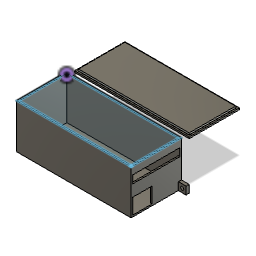
Sprinkler Case v5 (Autodesk Fusion 360 design; units mm, degrees)
Autodesk Fusion 360 part; units mm, degrees
sketch "Sketch1" plane through (0, 0, 0) normal (0, 1, 0) x (1, 0, 0)
  line L0 (0, 0) -> (145, 0)
  line L1 (0, 0) -> (0, -58)
  line L2 (0, -58) -> (145, -58)
  line L3 (145, -58) -> (145, 0)
  line L4 (145, 0) -> (0, 0)
  line L5 (0, 0) -> (0, -58)
  line L6 (0, 0) -> (-1.5, 0)
  line L7 (-1.5, 0) -> (-1.5, 1.5)
  line L8 (-1.5, 1.5) -> (0, 1.5)
  line L9 (0, 1.5) -> (0, 0)
  line L10 (145, -58) -> (146.5, -58)
  line L11 (146.5, -58) -> (146.5, -59.5)
  line L12 (146.5, -59.5) -> (145, -59.5)
  line L13 (145, -59.5) -> (145, -58)
  line L14 (-1.5, 1.5) -> (146.5, 1.5)
  line L15 (146.5, 1.5) -> (146.5, -59.5)
  line L16 (146.5, -59.5) -> (-1.5, -59.5)
  line L17 (-1.5, -59.5) -> (-1.5, 1.5)
  line L18 (146.5, 1.5) -> (148.5, 1.5)
  line L19 (148.5, 1.5) -> (148.5, 3.5)
  line L20 (148.5, 3.5) -> (146.5, 3.5)
  line L21 (146.5, 3.5) -> (146.5, 1.5)
  line L22 (-1.5, -59.5) -> (-3.5, -59.5)
  line L23 (-3.5, -59.5) -> (-3.5, -61.5)
  line L24 (-3.5, -61.5) -> (-1.5, -61.5)
  line L25 (-1.5, -61.5) -> (-1.5, -59.5)
  line L26 (-3.5, -61.5) -> (148.5, -61.5)
  line L27 (148.5, -61.5) -> (148.5, 3.5)
  line L28 (148.5, 3.5) -> (-3.5, 3.5)
  line L29 (-3.5, 3.5) -> (-3.5, -61.5)
  dimension "d7" = 145
  dimension "d8" = 58
  dimension "d9" = 1.5
  dimension "d10" = 1.5
  dimension "d11" = 1.5
  dimension "d12" = 1.5
  dimension "d13" = 2
  dimension "d14" = 2
  dimension "d15" = 2
  dimension "d16" = 2
  constraint coincident L0.start L1.start
  constraint horizontal L0
  constraint perpendicular L0 L1
  constraint horizontal L2
  constraint vertical L3
  constraint horizontal L4
  constraint vertical L5
  constraint horizontal L6
  constraint vertical L7
  constraint horizontal L8
  constraint vertical L9
  constraint horizontal L10
  constraint vertical L11
  constraint horizontal L12
  constraint vertical L13
  constraint horizontal L14
  constraint vertical L15
  constraint horizontal L16
  constraint vertical L17
  constraint horizontal L18
  constraint vertical L19
  constraint horizontal L20
  constraint vertical L21
  constraint horizontal L22
  constraint vertical L23
  constraint horizontal L24
  constraint vertical L25
  constraint horizontal L26
  constraint vertical L27
  constraint horizontal L28
  constraint vertical L29
  measures "d7" distance of L0.start L0.end
  measures "d8" distance of L0.start L1.end
  measures "d9" distance of L0.start L6.end
  measures "d10" distance of L0.start L8.end
  measures "d11" distance of L2.end L10.end
  measures "d12" distance of L2.end L12.end
  measures "d13" distance of L14.end L18.end
  measures "d14" distance of L14.end L20.end
  measures "d15" distance of L16.end L22.end
  measures "d16" distance of L16.end L24.end
extrude "Extrude1" add sketch "Sketch1" against normal blind 2 makes body 1
extrude "Extrude2" add sketch "Sketch1" along normal blind 55 contours L7 L8 L14 L17 L21 L22 L28 L29 | L22 L23 L24 L25 L26 L29 | L11 L12 L15 L16 L18 L25 L26 L27 | L18 L19 L20 L21 L27 L28 bodies 1
sketch "Sketch2" plane through (148.5, 0, 0) normal (1, 0, 0) x (0, 0, -1)
  line L0 (0, 0) -> (3.5, 0)
  line L1 (3.5, 0) -> (3.5, -2)
  line L2 (3.5, -2) -> (0, -2)
  line L3 (0, -2) -> (0, 0)
  line L4 (3.5, -2) -> (-61.5, -2)
  line L5 (-61.5, -2) -> (-61.5, 55)
  line L6 (-61.5, 55) -> (3.5, 55)
  line L7 (3.5, 55) -> (3.5, -2)
  line L8 (3.5, -2) -> (-61.5, -2)
  line L9 (-61.5, -2) -> (-61.5, 0)
  line L10 (-61.5, 0) -> (3.5, 0)
  line L11 (3.5, 0) -> (3.5, -2)
  line L12 (3.5, -2) -> (1.5, -2)
  line L13 (1.5, -2) -> (1.5, 55)
  line L14 (1.5, 55) -> (3.5, 55)
  line L15 (3.5, 55) -> (3.5, -2)
  line L16 (-61.5, -2) -> (-59.5, -2)
  line L17 (-59.5, -2) -> (-59.5, 55)
  line L18 (-59.5, 55) -> (-61.5, 55)
  line L19 (-61.5, 55) -> (-61.5, -2)
  line L20 (-59.5, 0) -> (-34.5, 0)
  line L21 (-34.5, 0) -> (-34.5, 20)
  line L22 (-34.5, 20) -> (-59.5, 20)
  line L23 (-59.5, 20) -> (-59.5, 0)
  line L24 (-59.5, 0) -> (-59.5, 45)
  line L25 (-59.5, 45) -> (1.5, 45)
  line L26 (1.5, 45) -> (1.5, 55)
  line L27 (1.5, 55) -> (-59.5, 55)
  line L28 (-59.5, 55) -> (-59.5, 45)
  line L29 (-59.5, 45) -> (1.5, 45)
  line L30 (1.5, 45) -> (1.5, 35)
  line L31 (1.5, 35) -> (-59.5, 35)
  line L32 (-59.5, 35) -> (-59.5, 45)
  dimension "d21" = 3.5
  dimension "d22" = 2
  dimension "d23" = 65
  dimension "d24" = 57
  dimension "d25" = 65
  dimension "d26" = 2
  dimension "d27" = 2
  dimension "d28" = 57
  dimension "d29" = 2
  dimension "d30" = 57
  dimension "d31" = 25
  dimension "d32" = 20
  dimension "d33" = 45
  dimension "d34" = 10
  constraint horizontal L0
  constraint vertical L1
  constraint horizontal L2
  constraint vertical L3
  constraint coincident L0.start L3.end
  constraint horizontal L4
  constraint vertical L5
  constraint horizontal L6
  constraint vertical L7
  constraint horizontal L8
  constraint vertical L9
  constraint horizontal L10
  constraint vertical L11
  constraint horizontal L12
  constraint vertical L13
  constraint horizontal L14
  constraint vertical L15
  constraint horizontal L16
  constraint vertical L17
  constraint horizontal L18
  constraint vertical L19
  constraint horizontal L20
  constraint vertical L21
  constraint horizontal L22
  constraint vertical L23
  constraint coincident L10 L20.start
  constraint coincident L17 L20.start
  constraint perpendicular L10 L24
  constraint horizontal L25
  constraint vertical L26
  constraint horizontal L27
  constraint vertical L28
  constraint horizontal L29
  constraint vertical L30
  constraint horizontal L31
  constraint vertical L32
  constraint coincident L13 L30.end
  measures "d21" distance of L0.start L0.end
  measures "d22" distance of L0.start L2.end
  measures "d23" distance of L1.end L4.end
  measures "d24" distance of L1.end L6.end
  measures "d25" distance of L1.end L4.end
  measures "d26" distance of L1.end L0.end
  measures "d27" distance of L1.end L12.end
  measures "d28" distance of L1.end L6.end
  measures "d29" distance of L4.end L16.end
  measures "d30" distance of L4.end L5.end
  measures "d31" distance of L20.start L20.end
  measures "d32" distance of L20.start L22.end
  measures "d33" distance of L20.start L24.end
  measures "d34" distance of L24.end L31.end
extrude "Extrude3" cut sketch "Sketch2" against normal blind 2 contours L10 L17 L20 L21 L22 L23 L24 | L13 L17 L24 L25 L29 L30 L31 L32 bodies 1
split "Split1" by plane through (146.5, 0, -1.5) normal (-1, 0, 0) bodies 1 makes body 2 at (96.5, -2, 39.8333)
ref_plane "WorkPlane1" through (142.5, 26.5, 29) normal (-1, 0, 0) x (0, 0, 1)
split "Split2" by plane through (142.5, 26.5, 29) normal (-1, 0, 0) bodies 2 makes body 3 at (93.8333, -2, 39.8333)
move_body "Move1" bodies 2 to x (1, 0, 0) y (0, 1, 0) z (0, 0, 1) at (0, 0, 85)
move_body "Move2" bodies 1 to x (1, 0, 0) y (0, 1, 0) z (0, 0, 1) at (-4, 0, 0)
combine "Combine1" operation add target body 3 tool bodies 1
sketch "Sketch3" plane through (0, 55, 0) normal (0, 1, 0) x (-1, 0, 0)
  line L0 (0, 0) -> (3.5, 0)
  line L1 (3.5, 0) -> (3.5, -3.5)
  line L2 (3.5, -3.5) -> (0, -3.5)
  line L3 (0, -3.5) -> (0, 0)
  line L4 (0, 0) -> (1.5, 0)
  line L5 (1.5, 0) -> (1.5, -1.5)
  line L6 (1.5, -1.5) -> (0, -1.5)
  line L7 (0, -1.5) -> (0, 0)
  line L8 (1.5, -1.5) -> (-142.5, -1.5)
  line L9 (-142.5, -1.5) -> (-142.5, 59.5)
  line L10 (-142.5, 59.5) -> (1.5, 59.5)
  line L11 (1.5, 59.5) -> (1.5, -1.5)
  line L12 (-142.5, 59.5) -> (-144.5, 59.5)
  line L13 (-144.5, 59.5) -> (-144.5, 61.5)
  line L14 (-144.5, 61.5) -> (-142.5, 61.5)
  line L15 (-142.5, 61.5) -> (-142.5, 59.5)
  line L16 (3.5, -3.5) -> (-144.5, -3.5)
  line L17 (-144.5, -3.5) -> (-144.5, 61.5)
  line L18 (-144.5, 61.5) -> (3.5, 61.5)
  line L19 (3.5, 61.5) -> (3.5, -3.5)
  dimension "d38" = 3.5
  dimension "d39" = 3.5
  dimension "d40" = 144
  dimension "d41" = 61
  dimension "d42" = 2
  dimension "d43" = 2
  constraint horizontal L0
  constraint vertical L1
  constraint horizontal L2
  constraint vertical L3
  constraint coincident L0.start L3.end
  constraint horizontal L4
  constraint vertical L5
  constraint horizontal L6
  constraint vertical L7
  constraint horizontal L8
  constraint vertical L9
  constraint horizontal L10
  constraint vertical L11
  constraint horizontal L12
  constraint vertical L13
  constraint horizontal L14
  constraint vertical L15
  constraint horizontal L16
  constraint vertical L17
  constraint horizontal L18
  constraint vertical L19
  measures "d38" distance of L0.start L0.end
  measures "d39" distance of L0.start L2.end
  measures "d40" distance of L5.end L8.end
  measures "d41" distance of L5.end L10.end
  measures "d42" distance of L9.end L12.end
  measures "d43" distance of L9.end L14.end
extrude "Extrude4" add sketch "Sketch3" along normal blind 2 separate body makes body 4
extrude "Extrude5" add sketch "Sketch3" against normal blind 2 separate body contours L0 L3 L4 L7 L8 L9 L10 L11 | L0 L3 L4 L5 L6 L7 L8 L11 makes body 5
combine "Combine2" operation add target body 4 tool bodies 5
chamfer "Chamfer1" distance 0.5 distance2 1.75 1 faces at (46.5, 53, 18.8333) on bodies 4
sketch "Sketch4" plane through (144.5, 0, 0) normal (1, 0, 0) x (0, 0, -1)
  line L0 (3.5, -2) -> (-0.5, -2)
  line L1 (-0.5, -2) -> (-0.5, 8)
  line L2 (-0.5, 8) -> (3.5, 8)
  line L3 (3.5, 8) -> (3.5, -2)
  dimension "d50" = 4
  dimension "d51" = 10
  constraint horizontal L0
  constraint vertical L1
  constraint horizontal L2
  constraint vertical L3
  measures "d50" distance of L0.start L0.end
  measures "d51" distance of L0.start L2.end
extrude "Extrude6" add sketch "Sketch4" along normal blind 10 bodies 3
sketch "Sketch5" plane through (-3.5, 0, 0) normal (-1, 0, 0) x (0, 0, 1)
  line L0 (-3.5, -2) -> (0.5, -2)
  line L1 (0.5, -2) -> (0.5, 8)
  line L2 (0.5, 8) -> (-3.5, 8)
  line L3 (-3.5, 8) -> (-3.5, -2)
  dimension "d54" = 4
  dimension "d55" = 10
  constraint horizontal L0
  constraint vertical L1
  constraint horizontal L2
  constraint vertical L3
  measures "d54" distance of L0.start L0.end
  measures "d55" distance of L0.start L2.end
extrude "Extrude7" add sketch "Sketch5" along normal blind 10 bodies 3
sketch "Sketch6" plane through (0, 0, 0.5) normal (0, 0, 1) x (1, 0, 0)
  line L0 (-3.5, -2) -> (-13.5, -2)
  line L1 (-13.5, -2) -> (-13.5, 8)
  line L2 (-13.5, 8) -> (-3.5, 8)
  line L3 (-3.5, 8) -> (-3.5, -2)
  line L4 (-3.5, -2) -> (-8.5, -2)
  line L5 (-8.5, -2) -> (-8.5, 3)
  line L6 (-8.5, 3) -> (-3.5, 3)
  line L7 (-3.5, 3) -> (-3.5, -2)
  circle A0 centre (-8.5, 3) radius 2
  dimension "d58" = 10
  dimension "d59" = 10
  dimension "d60" = 5
  dimension "d61" = 5
  dimension "d62" = 4
  constraint horizontal L0
  constraint vertical L1
  constraint horizontal L2
  constraint vertical L3
  constraint horizontal L4
  constraint vertical L5
  constraint horizontal L6
  constraint vertical L7
  constraint coincident L5.end L6.start
  measures "d58" distance of L0.start L0.end
  measures "d59" distance of L0.start L2.end
  measures "d60" distance of L0.start L4.end
  measures "d61" distance of L0.start L6.end
  measures "d62" diameter of A0
extrude "Extrude8" cut sketch "Sketch6" against normal blind 4 contours L5 L6 A0 | L5 L6 A0 bodies 3
sketch "Sketch7" plane through (0, 0, 0.5) normal (0, 0, 1) x (1, 0, 0)
  line L0 (144.5, -2) -> (154.5, -2)
  line L1 (154.5, -2) -> (154.5, 8)
  line L2 (154.5, 8) -> (144.5, 8)
  line L3 (144.5, 8) -> (144.5, -2)
  line L4 (144.5, -2) -> (149.5, -2)
  line L5 (149.5, -2) -> (149.5, 3)
  line L6 (149.5, 3) -> (144.5, 3)
  line L7 (144.5, 3) -> (144.5, -2)
  circle A0 centre (149.5, 3) radius 2
  dimension "d65" = 10
  dimension "d66" = 10
  dimension "d67" = 5
  dimension "d68" = 5
  dimension "d69" = 4
  constraint horizontal L0
  constraint vertical L1
  constraint horizontal L2
  constraint vertical L3
  constraint horizontal L4
  constraint vertical L5
  constraint horizontal L6
  constraint vertical L7
  constraint coincident L5.end L6.start
  measures "d65" distance of L0.start L0.end
  measures "d66" distance of L0.start L2.end
  measures "d67" distance of L0.start L4.end
  measures "d68" distance of L0.start L6.end
  measures "d69" diameter of A0
extrude "Extrude9" cut sketch "Sketch7" against normal blind 4 contours L5 L6 A0 | L5 L6 A0 bodies 3
move_body "Move3" bodies 4 to x (1, 0, 0) y (0, -1, 0) z (0, 0, -1) at (0, 106, -17)
delete_body "RemoveBody1" bodies 2
